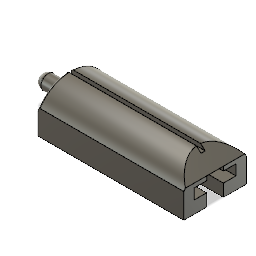
touch_test_gripper (Autodesk Fusion 360 design; units mm, degrees)
Autodesk Fusion 360 part; units mm, degrees
sketch "Sketch1" plane through (0, 0, 0) normal (0, 1, 0) x (1, 0, 0)
  line L0 (17.5, 7.5) -> (-17.5, 7.5)
  line L1 (-17.5, 7.5) -> (-17.5, -7.5)
  line L2 (-17.5, -7.5) -> (17.5, -7.5)
  line L3 (17.5, -7.5) -> (17.5, 7.5)
  line L4 (17.5, 7.5) -> (-17.5, -7.5) construction
  line L5 (-17.5, 7.5) -> (17.5, -7.5) construction
  dimension "d3" = 35
  dimension "d4" = 15
  constraint horizontal L0
  constraint perpendicular L0 L1
  constraint parallel L0 L2
  constraint parallel L1 L3
  constraint coincident L4 origin
  constraint coincident L5 origin
  measures "d3" distance of L1.end L2.end
  measures "d4" distance of L0.end L1.end
extrude "Extrude1" add sketch "Sketch1" along normal blind 10
sketch "Sketch2" plane through (17.5, 0, 0) normal (1, 0, 0) x (0, 0, -1)
  line L0 (-7.5, 0) -> (7.5, 0)
  line L1 (7.5, 0) -> (7.5, 10)
  line L2 (7.5, 10) -> (-7.5, 10)
  line L3 (-7.5, 10) -> (-7.5, 0)
  line L4 (-2, 0) -> (2, 0)
  line L5 (-2, 0) -> (-2, 3)
  line L6 (2, 0) -> (2, 3)
  line L7 (-2, 3) -> (-5, 3)
  line L8 (-5, 3) -> (-5, 5.5)
  line L9 (-5, 5.5) -> (-2, 5.5)
  line L10 (-2, 5.5) -> (-2, 6.5)
  line L11 (-2, 6.5) -> (2, 6.5)
  line L12 (2, 6.5) -> (2, 5.5)
  line L13 (2, 5.5) -> (5, 5.5)
  line L14 (5, 5.5) -> (5, 3)
  line L15 (5, 3) -> (2, 3)
  arc A0 (7.5, 6) -> (-7.5, 6) centre (0, 0.9687) ccw
  line L16 (-7.5, 6) -> (-7.5, 10)
  line L17 (7.5, 6) -> (7.5, 10)
  line L18 (7.5, 10) -> (-7.5, 10)
  dimension "d7" = 4
  dimension "d8" = 3
  dimension "d9" = 3
  dimension "d10" = 3
  dimension "d11" = 2.5
  dimension "d12" = 3
  dimension "d13" = 1
  dimension "d14" = 4
  dimension "d15" = 1
  dimension "d16" = 3
  dimension "d17" = 2.5
  dimension "d18" = 3
  dimension "d23" = 15
  dimension "d24" = 6
  constraint coincident L0 L4.start
  constraint parallel L0 L4
  constraint midpoint origin L4
  constraint perpendicular L0 L5
  constraint perpendicular L4 L6
  constraint perpendicular L5 L7
  constraint perpendicular L7 L8
  constraint perpendicular L8 L9
  constraint perpendicular L9 L10
  constraint perpendicular L10 L11
  constraint perpendicular L11 L12
  constraint perpendicular L12 L13
  constraint perpendicular L13 L14
  constraint perpendicular L14 L15
  constraint coincident L3 A0.end
  constraint coincident L2.end L3.start
  constraint coincident L1.end L2.start
  constraint perpendicular L2 L17
  measures "d7" distance of L4.start L4.end
  measures "d8" distance of L4.start L5.end
  measures "d9" distance of L4.end L6.end
  measures "d10" distance of L5.end L7.end
  measures "d11" distance of L7.end L8.end
  measures "d12" distance of L8.end L9.end
  measures "d13" distance of L9.end L10.end
  measures "d14" distance of L10.end L11.end
  measures "d15" distance of L11.end L12.end
  measures "d16" distance of L12.end L13.end
  measures "d17" distance of L13.end L14.end
  measures "d18" distance of L14.end L6.end
  measures "d23" distance of A0.end A0.start
  measures "d24" distance of L0.start A0.end
extrude "Extrude2" cut sketch "Sketch2" against normal blind 33 contours L0 L4 L5 L6 L7 L8 L9 L10 L11 L12 L13 L14 L15
extrude "Extrude3" cut sketch "Sketch2" against normal blind 35 contours L2 L3 A0 L16 L18 | L1 L2 A0 L17 L18
sketch "Sketch3" plane through (0, 0, 0) normal (0, 0, 1) x (1, 0, 0)
  line L0 (17.5, 6.5) -> (13.5, 10)
  line L1 (13.5, 10) -> (17.5, 10)
  line L2 (17.5, 10) -> (17.5, 6.5)
  point P0 (17.5, 0)
  dimension "d28" = 6.5
  constraint perpendicular L1 L2
  measures "d28" distance of L0.start P0
extrude "Extrude4" cut sketch "Sketch3" along normal blind 7.5 and the other way blind 7.5
fillet "Fillet1" radius 0.5 1 edges at (-17.5, 10, 0)
sketch "Sketch4" plane through (-17.5, 0, 0) normal (-1, 0, 0) x (0, 0, 1)
  arc A0 (7.5, 5.0347) -> (-7.5, 5.0347) centre (0, 0.9688) ccw
  line L0 (-7.5, 5.0347) -> (-7.5, 0)
  line L1 (-7.5, 0) -> (7.5, 0)
  line L2 (7.5, 0) -> (7.5, 5.0347)
  circle A1 centre (0, 5) radius 1.75
  circle A2 centre (0, 5) radius 1.25
  dimension "d36" = 3.5
  dimension "d38" = 2.5
  constraint concentric A1 A2
  measures "d36" diameter of A1
  measures "d38" diameter of A2
extrude "Extrude5" add sketch "Sketch4" along normal blind 5 contours A1 | A2
extrude "Extrude6" cut sketch "Sketch4" along normal blind 0.5 contours A1
sketch "Sketch6" plane through (0, 0, 0) normal (0, 0, 1) x (1, 0, 0)
  line L0 (-22.5, 6.75) -> (-22.5, 5)
  line L1 (-22.5, 5) -> (-24.25, 5)
  arc A0 (-22.5, 6.75) -> (-24.25, 5) centre (-22.5, 5) ccw
  dimension "d46" = 1.75
  constraint vertical L0
  constraint perpendicular L0 L1
  constraint coincident L0.end L1.start
  measures "d46" distance of L0.end L1.end
revolve "Revolve1" add sketch "Sketch6" angle 360 about axis through (-22.5, 5, 0) along (-1, 0, 0)
sketch "Sketch7" plane through (-17.5, 0, 0) normal (-1, 0, 0) x (0, 0, 1)
  circle A0 centre (0, 5) radius 1.25
  arc A1 (7.5, 5.0347) -> (-7.5, 5.0347) centre (0, 0.9688) ccw
  line L0 (-7.5, 5.0347) -> (-7.5, 0)
  line L1 (-7.5, 0) -> (7.5, 0)
  line L2 (7.5, 0) -> (7.5, 5.0347)
  line L3 (-0.5, 10) -> (-0.5, 5)
  line L4 (-0.5, 10) -> (0.5, 10)
  line L5 (0.5, 10) -> (0.5, 5)
  line L6 (-0.5, 5) -> (0.5, 5)
  dimension "d48" = 1
  dimension "d49" = 5
  constraint vertical L3
  constraint horizontal L4
  constraint perpendicular L4 L5
  measures "d48" distance of L3.start L4.end
  measures "d49" distance of L4.end L5.end
extrude "Extrude7" cut sketch "Sketch7" against normal blind 1 contours A0 L3 L5 L6 | A0 A1 L3 L5 | A1 L3 L4 L5 picked at (0, 5.4167)
sketch "Sketch8" plane through (-16.5, 0, 0) normal (-1, 0, 0) x (0, 0, 1)
  arc A0 (0.5, 9.9861) -> (-0.5, 9.9861) centre (0, 0.9687) ccw
  line L0 (-0.5, 9.9861) -> (-0.5, 5)
  line L1 (-0.5, 5) -> (0.5, 5)
  line L2 (0.5, 5) -> (0.5, 9.9861)
  line L3 (-0.5, 10) -> (0.5, 10)
  line L4 (0.5, 10) -> (0.5, 9)
  line L5 (0.5, 9) -> (-0.5, 9)
  line L6 (-0.5, 9) -> (-0.5, 10)
  constraint horizontal L3
  constraint vertical L4
  constraint horizontal L5
  constraint vertical L6
extrude "Extrude8" cut sketch "Sketch8" against normal blind 35 contours A0 L0 L2 L4 L5 L6
